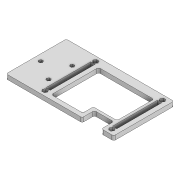
# Autodesk Inventor part: Middle PMMA
Saved by Autodesk Inventor 2020 (Build 240168000, 168)
## iProperties
Created: 2021-07-01
Part Number: Middle PMMA
Material: Generic
Document SubType Name: Modeling
Designer: ferrerx
Density: 1 g/cm^3
Appearance: Default
Author: ferrerx
Autodesk Inventor part; units mm, degrees
ref_plane "YZ Plane" through (0, 0, 0) normal (1, 0, 0) x (0, 1, 0)
ref_plane "XZ Plane" through (0, 0, 0) normal (0, 1, 0) x (-1, 0, 0)
ref_plane "XY Plane" through (0, 0, 0) normal (0, 0, 1) x (1, 0, 0)
sketch "Sketch1" plane through (0, 0, 0) normal (0, 1, 0) x (-1, 0, 0)
  line L0 (-2.27, 0) -> (120.44, 0)
  line L1 (120.44, 0) -> (120.44, -68.57)
  line L2 (120.44, -68.57) -> (-2.27, -68.57)
  line L3 (-2.27, -68.57) -> (-2.27, 0)
  line L4 (120.44, -66.57) -> (120.44, -2)
  line L5 (0, -68.57) -> (118.44, -68.57)
  line L6 (-2.27, -2.27) -> (-2.27, -66.3)
  circle A0 centre (81.55, -63.09) radius 1.5
  circle A1 centre (81.55, -63.09) radius 1.5
  line L7 (70.44, -68.57) -> (15.73, -68.57)
  line L8 (51, 0) -> (75, 0)
  line L9 (26, 0) -> (51, 0)
  line L10 (84, -60) -> (79, -60)
  line L11 (79, -60) -> (79, -8.7337)
  line L12 (79, -8.7337) -> (84, -8.7337)
  line L13 (84, -8.7337) -> (84, -60)
  line L14 (8, -60) -> (3, -60)
  line L15 (3, -60) -> (3, -8.7337)
  line L16 (3, -8.7337) -> (8, -8.7337)
  line L17 (8, -8.7337) -> (8, -60)
  circle A2 centre (5.25, -63.09) radius 1.5
  circle A3 centre (5.35, -5.47) radius 1.5
  circle A4 centre (81.55, -5.47) radius 1.5
  circle A5 centre (81.55, -5.47) radius 1.5
  circle A6 centre (5.35, -5.47) radius 1.5
  circle A7 centre (5.25, -63.09) radius 1.5
  dimension "d20" = 3
  dimension "d27" = 3
  dimension "d28" = 3
  dimension "d29" = 3
  dimension "d30" = 68.57
  constraints: 36 end point, 8 centre point, 6 parallel, 4 collinear, 4 concentric, 4 horizontal, 3 perpendicular, 3 point on line
  measures "d20" diameter of A0
  measures "d27" diameter of A2
  measures "d28" diameter of A3
  measures "d29" diameter of A4
  measures "d30" distance of L0.end L1.end
extrude "Extrusion1" add sketch "Sketch1" along normal blind 5
fillet "Fillet4" radius 2 4 edges at (-120.44, 2.5, -68.57) (-120.44, 2.5, 0) (2.27, 2.5, -68.57) (2.27, 2.5, 0)
sketch "Sketch7" plane through (0, 5, 0) normal (0, 1, 0) x (1, 0, 0)
  line L0 (-117.44, 63.57) -> (-87.44, 63.57)
  line L1 (-87.44, 63.57) -> (-87.44, 5)
  line L2 (-87.44, 5) -> (-117.44, 5)
  line L3 (-117.44, 5) -> (-117.44, 63.57)
  line L4 (-120.44, 66.57) -> (-120.44, 2) projected
  line L5 (0.27, 68.57) -> (-118.44, 68.57) projected
  line L6 (-118.44, 0) -> (0.27, 0) projected
  point P0 (0, 0)
  dimension "d67" = 30
  dimension "d68" = 3
  dimension "d69" = 5
  dimension "d70" = 5
  constraints: 8 end point, 2 parallel, 1 horizontal, 1 perpendicular
  measures "d67" distance of L1.end L2.end
  measures "d68" distance between parallel lines of L4 L3
  measures "d69" distance between parallel lines of L5 L0
  measures "d70" distance between parallel lines of L6 L2
extrude "Extrusion6" [suppressed]
fillet "Fillet8" [suppressed]
sketch "Sketch8" plane through (0, 5, 0) normal (0, 1, 0) x (1, 0, 0)
  line L0 (-118.44, 0) -> (0.27, 0) projected
  line L1 (-33.73, 0) -> (-11.73, 0)
  line L2 (-11.73, 0) -> (-11.73, 14)
  line L3 (-11.73, 14) -> (-33.73, 14)
  line L4 (-33.73, 14) -> (-33.73, 0)
  line L5 (2.27, 2) -> (2.27, 66.57) projected
  point P0 (0, 0)
  point P1 (-11.73, 0)
  dimension "d74" = 22
  dimension "d75" = 14
  dimension "d82" = 14
  constraints: 8 end point, 2 parallel, 1 horizontal, 1 perpendicular, 1 point on line
  measures "d74" distance between parallel lines of L2 L4
  measures "d75" distance of L3.end L1.start
  measures "d82" distance between parallel lines of L5 L2
extrude "Extrusion7" cut sketch "Sketch8" against normal blind 10
sketch "Sketch9" plane through (0, 5, 0) normal (0, 1, 0) x (1, 0, 0)
  line L0 (-74, 59) -> (-11, 59)
  line L1 (-11, 59) -> (-11, 17)
  line L2 (-11, 17) -> (-74, 17)
  line L3 (-74, 17) -> (-74, 59)
  line L4 (-74, 17) -> (-38, 17)
  line L5 (-38, 17) -> (-38, 5)
  line L6 (-38, 5) -> (-74, 5)
  line L7 (-74, 5) -> (-74, 17)
  point P0 (0, 0)
  constraints: 16 end point, 4 parallel, 2 horizontal, 2 perpendicular
extrude "Extrusion8" cut sketch "Sketch9" against normal blind 5
fillet "Fillet9" radius 2 6 edges at (-74, 2.5, -59) (-74, 2.5, -5) (-11, 2.5, -59) (-11, 2.5, -17) (-38, 2.5, -5) (-38, 2.5, -17)
fillet "Fillet10" radius 2 4 edges at (-33.73, 2.5, -14) (-11.73, 2.5, -14) (-11.73, 2.5, 0) (-33.73, 2.5, 0)
sketch "Sketch10" plane through (0, 0, 0) normal (0, -1, 0) x (1, 0, 0)
  circle A0 centre (-90.66, -18.55) radius 1
  circle A1 centre (-113.03, -32.07) radius 1
  circle A2 centre (-90.66, -45.53) radius 1
  line L0 (-120.44, -66.57) -> (-120.44, -2) projected
  line L1 (-118.44, 0) -> (-35.73, 0) projected
  line L2 (-90.66, -45.53) -> (-90.66, -18.55) construction
  point P0 (0, 0)
  dimension "d83" = 29.78
  dimension "d84" = 18.55
  dimension "d85" = 2
  dimension "d86" = 13.52
  dimension "d87" = 2
  dimension "d88" = 22.37
  dimension "d89" = 13.46
  dimension "d90" = 2
  constraints: 3 centre point, 2 end point, 1 vertical
  measures "d83" distance from line of L0 L2.end
  measures "d84" distance from line of L1 L2.end
  measures "d85" diameter of A0
  measures "d86" vertical distance of L2.end A1.centre
  measures "d87" diameter of A1
  measures "d88" horizontal distance of L2.end A1.centre
  measures "d89" vertical distance of A1.centre L2.start
  measures "d90" diameter of A2
extrude "Extrusion9" cut sketch "Sketch10" against normal blind 10
sketch "Sketch11" plane through (0, 0, 0) normal (0, -1, 0) x (1, 0, 0)
  circle A0 centre (-90.66, -18.55) radius 1 projected
  line L0 (-92.9694, -18.55) -> (-91.8147, -16.55)
  line L1 (-91.8147, -16.55) -> (-89.5053, -16.55)
  line L2 (-89.5053, -16.55) -> (-88.3506, -18.55)
  line L3 (-88.3506, -18.55) -> (-89.5053, -20.55)
  line L4 (-89.5053, -20.55) -> (-91.8147, -20.55)
  line L5 (-91.8147, -20.55) -> (-92.9694, -18.55)
  circle A1 centre (-113.03, -32.07) radius 1 projected
  line L6 (-115.3394, -32.07) -> (-114.1847, -30.07)
  line L7 (-114.1847, -30.07) -> (-111.8753, -30.07)
  line L8 (-111.8753, -30.07) -> (-110.7206, -32.07)
  line L9 (-110.7206, -32.07) -> (-111.8753, -34.07)
  line L10 (-111.8753, -34.07) -> (-114.1847, -34.07)
  line L11 (-114.1847, -34.07) -> (-115.3394, -32.07)
  circle A2 centre (-90.66, -45.53) radius 1 projected
  line L12 (-92.9694, -45.53) -> (-91.8147, -43.53)
  line L13 (-91.8147, -43.53) -> (-89.5053, -43.53)
  line L14 (-89.5053, -43.53) -> (-88.3506, -45.53)
  line L15 (-88.3506, -45.53) -> (-89.5053, -47.53)
  line L16 (-89.5053, -47.53) -> (-91.8147, -47.53)
  line L17 (-91.8147, -47.53) -> (-92.9694, -45.53)
  point P0 (0, 0)
  dimension "d93" = 4
  dimension "d94" = 4
  dimension "d95" = 4
  constraints: 36 end point, 3 coincident, 39 other
  measures "d93" distance between parallel lines of L16 L13
  measures "d94" distance between parallel lines of L7 L10
  measures "d95" distance between parallel lines of L4 L1
extrude "Extrusion10" cut sketch "Sketch11" against normal blind 10
sketch "Sketch12" plane through (0, 0, 0) normal (0, -1, 0) x (1, 0, 0)
  circle A0 centre (-5.35, -5.47) radius 1.5 projected
  line L0 (-8.2368, -5.47) -> (-6.7934, -2.97)
  line L1 (-6.7934, -2.97) -> (-3.9066, -2.97)
  line L2 (-3.9066, -2.97) -> (-2.4632, -5.47)
  line L3 (-2.4632, -5.47) -> (-3.9066, -7.97)
  line L4 (-3.9066, -7.97) -> (-6.7934, -7.97)
  line L5 (-6.7934, -7.97) -> (-8.2368, -5.47)
  circle A1 centre (-81.55, -5.47) radius 1.5 projected
  line L6 (-84.4368, -5.47) -> (-82.9934, -2.97)
  line L7 (-82.9934, -2.97) -> (-80.1066, -2.97)
  line L8 (-80.1066, -2.97) -> (-78.6632, -5.47)
  line L9 (-78.6632, -5.47) -> (-80.1066, -7.97)
  line L10 (-80.1066, -7.97) -> (-82.9934, -7.97)
  line L11 (-82.9934, -7.97) -> (-84.4368, -5.47)
  circle A2 centre (-81.55, -63.09) radius 1.5 projected
  line L12 (-84.4368, -63.09) -> (-82.9934, -60.59)
  line L13 (-82.9934, -60.59) -> (-80.1066, -60.59)
  line L14 (-80.1066, -60.59) -> (-78.6632, -63.09)
  line L15 (-78.6632, -63.09) -> (-80.1066, -65.59)
  line L16 (-80.1066, -65.59) -> (-82.9934, -65.59)
  line L17 (-82.9934, -65.59) -> (-84.4368, -63.09)
  circle A3 centre (-5.25, -63.09) radius 1.5 projected
  line L18 (-6.6934, -60.59) -> (-3.8066, -60.59)
  line L19 (-3.8066, -60.59) -> (-2.3632, -63.09)
  line L20 (-2.3632, -63.09) -> (-3.8066, -65.59)
  line L21 (-3.8066, -65.59) -> (-6.6934, -65.59)
  line L22 (-6.6934, -65.59) -> (-8.1368, -63.09)
  line L23 (-8.1368, -63.09) -> (-6.6934, -60.59)
  line L24 (-8, -60) -> (-3, -60) projected
  line L25 (-84, -60) -> (-79, -60) projected
  line L26 (-79, -8.7337) -> (-84, -8.7337) projected
  line L27 (-3, -8.7337) -> (-8, -8.7337) projected
  point P0 (0, 0)
  dimension "d98" = 5
  dimension "d99" = 5
  dimension "d100" = 5
  constraints: 48 end point, 4 coincident, 4 parallel, 1 point on line, 52 other
  measures "d98" distance between parallel lines of L21 L18
  measures "d99" distance between parallel lines of L7 L10
  measures "d100" distance between parallel lines of L1 L4
extrude "Extrusion11" cut sketch "Sketch12" against normal blind 10
body "Solid1"
